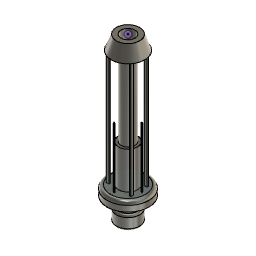
Buoyani-3D-v2 (Autodesk Fusion 360 design; units mm, degrees)
Autodesk Fusion 360 part; units mm, degrees
sketch "Sketch1" plane through (0, 0, 0) normal (0, 0, 1) x (1, 0, 0)
  circle A0 centre (0, 0) radius 25
  dimension "d1" = 50
  constraint coincident A0.centre origin
  measures "d1" diameter of A0
extrude "Extrude1" add sketch "Sketch1" along normal blind 20 makes body 1
extrude "Extrude2" add 1 faces at (-6.7759, -1.242, 20) along direction (0, 0, 1) blind 10 on bodies 1 bodies 1
fillet "Fillet1" radius 4.5 1 faces at (-24.8758, 2.4892, 10) on bodies 1
extrude "Extrude3" add 1 faces at (5.4025, 6.3711, 30) along direction (0, 0, 1) blind 20 on bodies 1 bodies 1
sketch "Sketch2" plane through (0, 0, 50) normal (0, 0, 1) x (-1, 0, 0)
  circle A0 centre (0, 0) radius 20.5
  circle A1 centre (0, 0) radius 45
  dimension "d9" = 90
  constraint coincident A0.centre A1.centre
  measures "d9" diameter of A1
extrude "Extrude4" add sketch "Sketch2" along normal blind 20 separate body makes body 2
extrude "Extrude5" add 1 faces at (5.4025, 6.3711, 50) along direction (0, 0, 1) blind 100 on bodies 1 bodies 1 2
fillet "Fillet2" radius 7.5 1 edges at (41.9547, 16.2727, 70) on bodies 1
sketch "Sketch3" plane through (0, 0, 70) normal (0, 0, 1) x (-1, 0, 0)
  circle A0 centre (0, 0) radius 20.5
  circle A1 centre (0, 0) radius 37.5
  line L0 (-1, -29) -> (1, -29)
  line L1 (1, -29) -> (1, -31)
  line L2 (1, -31) -> (-1, -31)
  line L3 (-1, -31) -> (-1, -29)
  line L4 (-1, -29) -> (1, -31) construction
  line L5 (1, -29) -> (-1, -31) construction
  point P0 (0, -30)
  dimension "d15" = 2
  constraint horizontal L0
  constraint perpendicular L0 L1
  constraint parallel L0 L2
  constraint parallel L1 L3
  constraint coincident L4 P0
  constraint coincident L5 P0
  measures "d15" distance of L1.end L2.end
extrude "Extrude6" add sketch "Sketch3" along normal blind 100 contours L0 L1 L2 L3 bodies 1
move_face "MoveFace1" to x (0.939693, -0.34202, 0) y (0.34202, 0.939693, 0) z (0, 0, 1) at (-10.0558, 1.1527, 0) 1 faces at (0.3333, 29.6667, 170) on bodies 1
move_face "MoveFace2" by (1, -1, 0) 1 faces at (0.3333, 29.6667, 170) on bodies 1
sketch "Sketch4" plane through (0, 0, 70) normal (0, 0, 1) x (-1, 0, 0)
  line L0 (-1, -31) -> (-1, -29)
  line L1 (-1, -29) -> (1, -29)
  line L2 (1, -29) -> (1, -31)
  line L3 (1, -31) -> (-1, -31)
  circle A0 centre (0, 0) radius 20.5
  circle A1 centre (0, 0) radius 37.5
  line L4 (-1, 29) -> (1, 29)
  line L5 (1, 29) -> (1, 31)
  line L6 (1, 31) -> (-1, 31)
  line L7 (-1, 31) -> (-1, 29)
  line L8 (-1, 29) -> (1, 31) construction
  line L9 (1, 29) -> (-1, 31) construction
  point P0 (0, 30)
  dimension "d18" = 2
  constraint horizontal L4
  constraint perpendicular L4 L5
  constraint parallel L4 L6
  constraint parallel L5 L7
  constraint coincident L8 P0
  constraint coincident L9 P0
  measures "d18" distance of L4.end L5.end
extrude "Extrude7" add sketch "Sketch4" along normal blind 10 contours L4 L5 L6 L7 bodies 1
extrude "Extrude8" add 1 faces at (0.3333, -30.3333, 80) along direction (0, 0, 1) blind 90 on bodies 1 bodies 1
sketch "Sketch5" plane through (0, 0, 70) normal (0, 0, 1) x (-1, 0, 0)
  line L0 (-1, 31) -> (1, 31)
  line L1 (1, 31) -> (1, 29)
  line L2 (1, 29) -> (-1, 29)
  line L3 (-1, 29) -> (-1, 31)
  line L4 (-1, -31) -> (-1, -29)
  line L5 (-1, -29) -> (1, -29)
  line L6 (1, -29) -> (1, -31)
  line L7 (1, -31) -> (-1, -31)
  circle A0 centre (0, 0) radius 20.5
  circle A1 centre (0, 0) radius 37.5
  line L8 (29, -1) -> (31, -1)
  line L9 (31, -1) -> (31, 1)
  line L10 (31, 1) -> (29, 1)
  line L11 (29, 1) -> (29, -1)
  line L12 (29, -1) -> (31, 1) construction
  line L13 (31, -1) -> (29, 1) construction
  point P0 (30, 0)
  dimension "d23" = 2
  constraint horizontal L8
  constraint perpendicular L8 L9
  constraint parallel L8 L10
  constraint parallel L9 L11
  constraint coincident L12 P0
  constraint coincident L13 P0
  measures "d23" distance of L9.end L10.end
extrude "Extrude9" add sketch "Sketch5" along normal blind 100 contours L8 L9 L10 L11 bodies 1
sketch "Sketch6" plane through (0, 0, 70) normal (0, 0, 1) x (-1, 0, 0)
  line L0 (29, 1) -> (31, 1)
  line L1 (31, 1) -> (31, -1)
  line L2 (31, -1) -> (29, -1)
  line L3 (29, -1) -> (29, 1)
  line L4 (-1, 31) -> (1, 31)
  line L5 (1, 31) -> (1, 29)
  line L6 (1, 29) -> (-1, 29)
  line L7 (-1, 29) -> (-1, 31)
  line L8 (-1, -31) -> (-1, -29)
  line L9 (-1, -29) -> (1, -29)
  line L10 (1, -29) -> (1, -31)
  line L11 (1, -31) -> (-1, -31)
  circle A0 centre (0, 0) radius 20.5
  circle A1 centre (0, 0) radius 37.5
  line L12 (-31, -1) -> (-29, -1)
  line L13 (-29, -1) -> (-29, 1)
  line L14 (-29, 1) -> (-31, 1)
  line L15 (-31, 1) -> (-31, -1)
  line L16 (-31, -1) -> (-29, 1) construction
  line L17 (-29, -1) -> (-31, 1) construction
  point P0 (-30, 0)
  dimension "d26" = 2
  constraint horizontal L12
  constraint perpendicular L12 L13
  constraint parallel L12 L14
  constraint parallel L13 L15
  constraint coincident L16 P0
  constraint coincident L17 P0
  measures "d26" distance of L13.end L14.end
extrude "Extrude10" add sketch "Sketch6" along normal blind 100 contours L12 L13 L14 L15 bodies 1
sketch "Sketch7" plane through (0, 0, 150) normal (0, 0, 1) x (-1, 0, 0)
  circle A0 centre (0, 0) radius 20.5
  circle A1 centre (0, 0) radius 15
  dimension "d29" = 30
  constraint coincident A0.centre A1.centre
  measures "d29" diameter of A1
extrude "Extrude11" add sketch "Sketch7" along normal blind 200 contours A1 bodies 1
box "BoxPrimitive1" add length 3 width 6 height 1 placed x (0, -1, 0) y (1, 0, 0) z (0, 0, 1) at (20, 18, 70) bodies 1
box "BoxPrimitive2" add length 6 width 3 height 1 placed x (0, -1, 0) y (1, 0, 0) z (0, 0, 1) at (-27, 18, 70) bodies 1
box "BoxPrimitive3" add length 3 width 6 height 1 placed x (0, 1, 0) y (-1, 0, 0) z (0, 0, 1) at (-21, -20, 70) bodies 1
sketch "Sketch11" plane through (0, 0, 70) normal (0, 0, 1) x (-1, 0, 0)
  line L0 (21, 17) -> (21, 20)
  line L1 (21, 20) -> (27, 20)
  line L2 (27, 20) -> (27, 17)
  line L3 (27, 17) -> (21, 17)
  line L4 (27, -12) -> (27, -18)
  line L5 (27, -18) -> (24, -18)
  line L6 (24, -18) -> (24, -12)
  line L7 (24, -12) -> (27, -12)
  line L8 (-20, -15) -> (-20, -18)
  line L9 (-20, -18) -> (-26, -18)
  line L10 (-26, -18) -> (-26, -15)
  line L11 (-26, -15) -> (-20, -15)
  line L12 (-31, 1) -> (-29, 1)
  line L13 (-29, 1) -> (-29, -1)
  line L14 (-29, -1) -> (-31, -1)
  line L15 (-31, -1) -> (-31, 1)
  line L16 (29, 1) -> (31, 1)
  line L17 (31, 1) -> (31, -1)
  line L18 (31, -1) -> (29, -1)
  line L19 (29, -1) -> (29, 1)
  line L20 (-1, 31) -> (1, 31)
  line L21 (1, 31) -> (1, 29)
  line L22 (1, 29) -> (-1, 29)
  line L23 (-1, 29) -> (-1, 31)
  line L24 (-1, -31) -> (-1, -29)
  line L25 (-1, -29) -> (1, -29)
  line L26 (1, -29) -> (1, -31)
  line L27 (1, -31) -> (-1, -31)
  circle A0 centre (0, 0) radius 20.5
  circle A1 centre (0, 0) radius 37.5
box "BoxPrimitive4" add length 6 width 3 height 1 placed x (0, 1, 0) y (-1, 0, 0) z (0, 0, 1) at (26, -20, 70) bodies 1
extrude "Extrude12" add 1 faces at (24, -18, 71) along direction (0, 0, 1) blind 250 on bodies 1 bodies 1
extrude "Extrude13" add 1 faces at (24, 17, 71) along direction (0, 0, 1) blind 250 on bodies 1 bodies 1
extrude "Extrude14" add 1 faces at (-25, -19, 71) along direction (0, 0, 1) blind 250 on bodies 1 bodies 1
extrude "Extrude15" add 1 faces at (-25, 16, 71) along direction (0, 0, 1) blind 250 on bodies 1 bodies 1
sketch "Sketch13" plane through (0, 0, 350) normal (0, 0, 1) x (-1, 0, 0)
  circle A0 centre (0, 0) radius 15
sketch "Sketch14" plane through (0, 0, 350) normal (0, 0, 1) x (-1, 0, 0)
extrude "Extrude16" cut sketch "Sketch13" against normal blind 30 bodies 1
sketch "Sketch15" plane through (0, 0, 320) normal (0, 0, 1) x (-1, 0, 0)
  circle A0 centre (0, 0) radius 15
  circle A1 centre (0, 0) radius 25
  dimension "d63" = 50
  constraint concentric A0 A1
  measures "d63" diameter of A1
extrude "Extrude17" add sketch "Sketch15" along normal blind 30 separate body makes body 3
draft "Draft1" angle 20 neutral plane through (0, 0, 350) pull (0, 0, 1) 1 faces at (24.8758, -2.4892, 330) on bodies 3
